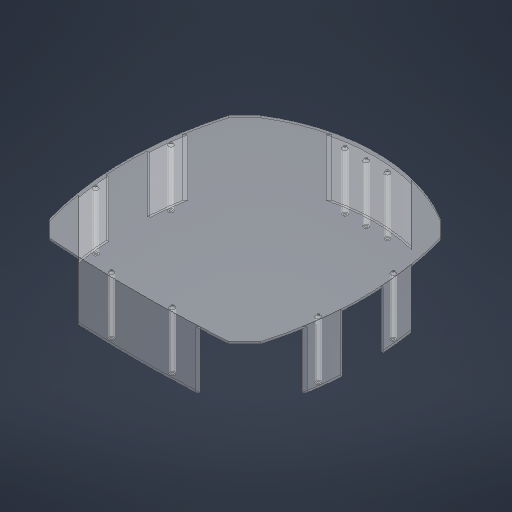
# Autodesk Inventor part: Spider_Robot_Chasis_Top_V1
Saved by Autodesk Inventor 2026.2 (Build 302298010, 298A)
## iProperties
Created: 2026-09-09
Part Number: Spider_Robot_Chasis_Top_V1
Material: Generic
Document SubType Name: Modeling
Designer: Entity
Density: 1 g/cm^3
Appearance: Clear - Light
Mass: 138.389 g
Surface Area: 1463.19 cm^2
Volume: 138.389 cm^3
Author: Entity
Autodesk Inventor part; units mm, degrees
ref_plane "YZ Plane" through (0, 0, 0) normal (1, 0, 0) x (0, 1, 0)
ref_plane "XZ Plane" through (0, 0, 0) normal (0, 1, 0) x (-1, 0, 0)
ref_plane "XY Plane" through (0, 0, 0) normal (0, 0, 1) x (1, 0, 0)
sketch "Sketch1" plane through (0, 0, 0) normal (0, 1, 0) x (-1, 0, 0)
  line L0 (11.257, 34.2721) -> (-44.743, 34.2721)
  line L1 (-44.743, 34.2721) -> (-44.743, -50.7279)
  line L2 (-44.743, -50.7279) -> (11.257, -50.7279)
  line L3 (11.257, -50.7279) -> (11.257, 34.2721)
  line L4 (-16.743, -50.7279) -> (-16.743, -57.7279)
  line L5 (14.507, -57.7279) -> (-47.993, -57.7279)
  line L6 (-47.993, -57.7279) -> (-47.993, -83.1279)
  line L7 (-47.993, -83.1279) -> (14.507, -83.1279)
  line L8 (14.507, -83.1279) -> (14.507, -57.7279)
  line L9 (-16.743, 34.2721) -> (-16.743, 41.2721)
  line L10 (-4.243, 41.2721) -> (-29.243, 41.2721)
  line L11 (-29.243, 41.2721) -> (-29.243, 51.2721)
  line L12 (-29.243, 51.2721) -> (-4.243, 51.2721)
  line L13 (-4.243, 51.2721) -> (-4.243, 41.2721)
  line L14 (-16.743, -83.1279) -> (-16.743, -90.1279)
  line L15 (23.257, -160.1279) -> (-56.743, -160.1279)
  line L16 (-56.743, -160.1279) -> (-56.743, -90.1279)
  line L17 (-56.743, -90.1279) -> (23.257, -90.1279)
  line L18 (23.257, -90.1279) -> (23.257, -160.1279)
  line L19 (14.507, -54.4279) -> (21.507, -54.4279)
  line L20 (14.507, -57.7279) -> (14.507, -54.4279)
  line L21 (46.907, -85.6779) -> (21.507, -85.6779)
  line L22 (21.507, -85.6779) -> (21.507, -23.1779)
  line L23 (21.507, -23.1779) -> (46.907, -23.1779)
  line L24 (46.907, -23.1779) -> (46.907, -85.6779)
  line L25 (-80.393, -85.6779) -> (-54.993, -85.6779)
  line L26 (-54.993, -85.6779) -> (-54.993, -23.1779)
  line L27 (-54.993, -23.1779) -> (-80.393, -23.1779)
  line L28 (-80.393, -23.1779) -> (-80.393, -85.6779)
  line L29 (-80.393, -54.4279) -> (-87.393, -54.4279)
  line L30 (-16.743, -160.1279) -> (-16.743, 51.2721)
  line L31 (-16.743, -54.4279) -> (63.257, -54.4279) construction
  line L32 (-16.743, -54.4279) -> (-69.7761, -107.4609)
  line L33 (-16.743, -54.4279) -> (58.257, -54.4279) construction
  line L34 (-69.7761, -107.4609) -> (-80.3827, -118.0675)
  line L35 (-80.3827, -118.0675) -> (-88.1608, -110.2893)
  line L36 (-88.1608, -110.2893) -> (-119.2735, -141.402)
  line L37 (-119.2735, -141.402) -> (-103.7172, -156.9584)
  line L38 (-103.7172, -156.9584) -> (-72.6045, -125.8457)
  line L39 (-72.6045, -125.8457) -> (-80.3827, -118.0675)
  line L40 (86.0976, -54.4279) -> (-151.9015, -54.4279)
  line L41 (-87.393, -54.4279) -> (-87.393, -65.4279)
  line L42 (-87.393, -65.4279) -> (-131.393, -65.4279)
  line L43 (-131.393, -65.4279) -> (-131.393, -43.4279)
  line L44 (-131.393, -43.4279) -> (-87.393, -43.4279)
  line L45 (-87.393, -43.4279) -> (-87.393, -54.4279)
  line L46 (-80.3827, 9.2117) -> (-88.1608, 1.4335)
  line L47 (-88.1608, 1.4335) -> (-119.2735, 32.5462)
  line L48 (-119.2735, 32.5462) -> (-103.7172, 48.1026)
  line L49 (-103.7172, 48.1026) -> (-72.6045, 16.9899)
  line L50 (-72.6045, 16.9899) -> (-80.3827, 9.2117)
  line L51 (46.8966, -118.0675) -> (54.6747, -110.2893)
  line L52 (54.6747, -110.2893) -> (85.7874, -141.402)
  line L53 (85.7874, -141.402) -> (70.2311, -156.9584)
  line L54 (70.2311, -156.9584) -> (39.1184, -125.8457)
  line L55 (39.1184, -125.8457) -> (46.8966, -118.0675)
  line L56 (53.907, -54.4279) -> (53.907, -65.4279)
  line L57 (53.907, -65.4279) -> (97.907, -65.4279)
  line L58 (97.907, -65.4279) -> (97.907, -43.4279)
  line L59 (97.907, -43.4279) -> (53.907, -43.4279)
  line L60 (53.907, -43.4279) -> (53.907, -54.4279)
  line L61 (54.6747, 1.4335) -> (85.7874, 32.5462)
  line L62 (85.7874, 32.5462) -> (70.2311, 48.1026)
  line L63 (70.2311, 48.1026) -> (39.1184, 16.9899)
  line L64 (46.8966, 9.2117) -> (54.6747, 1.4335)
  line L65 (39.1184, 16.9899) -> (46.8966, 9.2117)
  point P0 (-16.743, -57.7279)
  point P1 (-29.243, 46.2721)
  point P2 (-16.743, -90.1279)
  point P3 (21.507, -54.4279)
  point P4 (-83.893, -54.4279)
  point P5 (-54.993, -54.4279)
  point P6 (-44.743, -8.2279)
  point P7 (-87.393, -42.4279)
  dimension "d22" = 85
  dimension "d23" = 56
  dimension "d29" = 7
  dimension "d30" = 62.5
  dimension "d31" = 25.4
  dimension "d32" = 0
  dimension "d33" = 0
  dimension "d34" = 7
  dimension "d35" = 10
  dimension "d36" = 25
  dimension "d37" = 0
  dimension "d38" = 0
  dimension "d53" = 7
  dimension "d54" = 80
  dimension "d55" = 70
  dimension "d56" = 0
  dimension "d57" = 0
  dimension "d59" = 7
  dimension "d60" = 3.3
  dimension "d61" = 25.4
  dimension "d62" = 62.5
  dimension "d63" = 0
  dimension "d64" = 0
  dimension "d65" = 7
  dimension "d73" = 75
  dimension "d74" = 135
  dimension "d75" = 15
  dimension "d76" = 11
  dimension "d77" = 44
  dimension "d78" = 22
  dimension "d84" = 31.25
  dimension "d85" = 46.2
  dimension "d87" = 25.4
  dimension "d88" = 62.5
  dimension "d91" = 7
  dimension "d92" = 10.25
  dimension "d97" = 11
  dimension "d98" = 44
  dimension "d99" = 22
  constraints: 132 end point, 20 symmetric about line, 15 midpoint, 12 perpendicular, 10 parallel, 9 horizontal, 7 point on line, 5 vertical, 1 equal length
  measures "d22" distance of L0.end L1.end
  measures "d23" distance of L1.end L2.end
  measures "d29" distance of L4.start L4.end
  measures "d30" distance of L6.end L7.end
  measures "d31" distance of L5.end L6.end
  measures "d32" distance of L4.end point (-16.743, -57.728)
  measures "d33" distance of point (-16.743, -57.728) L4.end
  measures "d34" distance of L9.start L9.end
  measures "d35" distance of L12.end L10.start
  measures "d36" distance of L11.end L12.end
  measures "d37" distance of L9.end point (-16.743, 41.272)
  measures "d38" distance of L9.end point (-16.743, 41.272)
  measures "d53" distance of L14.start L14.end
  measures "d54" distance of L16.end L17.end
  measures "d55" distance of L15.end L16.end
  measures "d56" distance of L14.end point (-16.743, -90.128)
  measures "d57" distance of point (-16.743, -90.128) L14.end
  measures "d59" distance of L19.start L19.end
  measures "d60" distance of L5.start L19.start
  measures "d61" distance of L22.end L23.end
  measures "d62" distance of L21.end L22.end
  measures "d63" distance of L19.end point (21.507, -54.428)
  measures "d64" distance of point (21.507, -54.428) L19.end
  measures "d65" distance of L29.start L29.end
  measures "d73" distance of L31.start L32.end
  measures "d74" angle of L32 L33
  measures "d75" distance of L32.end L34.end
  measures "d76" distance of L34.end L35.end
  measures "d77" distance of L35.end L36.end
  measures "d78" distance of L36.end L37.end
  measures "d84" vertical distance of L28.start point (-83.893, -54.428)
  measures "d85" vertical distance of point (-54.993, -54.428) point (-44.743, -8.228)
  measures "d87" distance of L27.start L28.start
  measures "d88" distance of L25.end L27.start
  measures "d91" horizontal distance of L25.end L6.end
  measures "d92" horizontal distance of L27.start point (-44.743, -8.228)
  measures "d97" distance of L29.end L41.end
  measures "d98" distance of L41.end L42.end
  measures "d99" distance of L42.end L43.end
extrude "Extrusion1" add sketch "Sketch1" along normal blind 54 contours L3 L2 L30 L0 | L30 L2 L1 L0 | L30 L7 L32 L5 | L5 L8 L7 L30 | L32 L7 L6 L5 | L30 L15 L16 L32 L17 | L17 L18 L15 L30 | L32 L16 L17 | L10 L30 L12 L13 | L10 L11 L12 L30 | L21 L22 L40 L24 | L40 L22 L23 L24 | L28 L40 L26 L25 | L28 L27 L26 L40 | L39 L38 L37 L36 L35 | L41 L42 L43 L40 | L40 L43 L44 L45 | L46 L47 L48 L49 L50 | L51 L52 L53 L54 L55 | L60 L59 L58 L57 L56 | L64 L65 L63 L62 L61
sketch "Sketch2" plane through (0, 0, 0) normal (0, -1, 0) x (1, 0, 0)
  line L0 (56.743, -160.1279) -> (-23.257, -160.1279) projected
  line L1 (4.243, 51.2721) -> (29.243, 51.2721) projected
  line L2 (-85.7874, 32.5462) -> (-70.2311, 48.1026) projected
  line L3 (-70.2311, 48.1026) -> (-229.2278, -110.8941)
  line L4 (-70.2311, -156.9584) -> (-85.7874, -141.402) projected
  line L5 (-70.2311, -156.9584) -> (-201.5199, -25.6696)
  line L6 (103.7172, -156.9584) -> (72.6045, -125.8457) projected
  line L7 (103.7172, -156.9584) -> (295.0011, 34.3256)
  line L8 (103.7172, 48.1026) -> (119.2735, 32.5462) projected
  line L9 (103.7172, 48.1026) -> (277.6654, -125.8457)
  line L10 (103.7172, 48.1026) -> (-70.2311, 48.1026)
  arc A0 (-70.2311, -156.9584) -> (103.7172, -156.9584) centre (16.743, -16.5068) ccw
  line L11 (47.993, -83.1279) -> (-14.507, -83.1279) projected
  line L12 (16.743, -83.1279) -> (16.743, -57.7279)
  line L13 (-14.507, -57.7279) -> (47.993, -57.7279) projected
  arc A1 (103.7172, 48.1026) -> (-70.2311, 48.1026) centre (16.743, -1143.6334) ccw
  line L14 (-97.907, -65.4279) -> (-97.907, -43.4279) projected
  arc A2 (-85.7874, 32.5462) -> (-85.7874, -141.402) centre (215.2401, -54.4279) ccw
  line L15 (131.393, -43.4279) -> (131.393, -65.4279) projected
  arc A3 (119.2735, -141.402) -> (119.2735, 32.5462) centre (-181.754, -54.4279) ccw
  point P0 (0, 0)
  point P1 (-172.7616, -54.4279)
  dimension "d133" = 1194.9055
  dimension "d134" = 313.3402
  dimension "d135" = 313.3402
  dimension "d136" = 165.2003
  constraints: 12 end point, 10 point on circle, 4 centre point, 3 collinear, 2 midpoint, 1 horizontal, 1 perpendicular, 1 point on line
  measures "d133" radius of A1
  measures "d134" radius of A3
  measures "d135" radius of A2
  measures "d136" radius of A0
extrude "Extrusion2" add sketch "Sketch2" along normal blind 57 contours L2 L10 L8 A3 L15 L7 A0 L4 A2 L14 | A1 L10 | L14 A2 | A3 L15
sketch "Sketch11" plane through (0, 54, 0) normal (0, 1, 0) x (1, 0, 0)
  line L0 (56.743, 160.1279) -> (-23.257, 160.1279) projected
  line L1 (56.743, 90.1279) -> (56.743, 160.1279) projected
  line L2 (-23.257, 160.1279) -> (56.743, 160.1279)
  line L3 (56.743, 160.1279) -> (56.743, 90.1279)
  line L4 (56.743, 90.1279) -> (-23.257, 90.1279)
  line L5 (-23.257, 90.1279) -> (-23.257, 160.1279)
  line L6 (47.993, 83.1279) -> (-14.507, 83.1279) projected
  line L7 (-14.507, 57.7279) -> (47.993, 57.7279) projected
  line L8 (-14.507, 83.1279) -> (47.993, 83.1279)
  line L9 (47.993, 83.1279) -> (47.993, 57.7279)
  line L10 (47.993, 57.7279) -> (-14.507, 57.7279)
  line L11 (-14.507, 57.7279) -> (-14.507, 83.1279)
  line L12 (-21.507, 85.6779) -> (-46.907, 85.6779) projected
  line L13 (-21.507, 23.1779) -> (-21.507, 85.6779) projected
  line L14 (-46.907, 85.6779) -> (-21.507, 85.6779)
  line L15 (-21.507, 85.6779) -> (-21.507, 23.1779)
  line L16 (-21.507, 23.1779) -> (-46.907, 23.1779)
  line L17 (-46.907, 23.1779) -> (-46.907, 85.6779)
  line L18 (80.393, 23.1779) -> (80.393, 85.6779) projected
  line L19 (54.993, 23.1779) -> (80.393, 23.1779)
  line L20 (80.393, 23.1779) -> (80.393, 85.6779)
  line L21 (80.393, 85.6779) -> (54.993, 85.6779)
  line L22 (54.993, 85.6779) -> (54.993, 23.1779)
  line L23 (44.743, 50.7279) -> (-11.257, 50.7279) projected
  line L24 (-11.257, -34.2721) -> (44.743, -34.2721) projected
  line L25 (-11.257, 50.7279) -> (44.743, 50.7279)
  line L26 (44.743, 50.7279) -> (44.743, -34.2721)
  line L27 (44.743, -34.2721) -> (-11.257, -34.2721)
  line L28 (-11.257, -34.2721) -> (-11.257, 50.7279)
  line L29 (29.243, -41.2721) -> (4.243, -41.2721) projected
  line L30 (29.243, -51.2721) -> (29.243, -41.2721) projected
  line L31 (4.243, -41.2721) -> (29.243, -41.2721)
  line L32 (29.243, -41.2721) -> (29.243, -51.2721)
  line L33 (29.243, -51.2721) -> (4.243, -51.2721)
  line L34 (4.243, -51.2721) -> (4.243, -41.2721)
  line L35 (-54.6747, 110.2893) -> (-39.1184, 125.8457) projected
  line L36 (-54.6747, 110.2893) -> (-39.1184, 125.8457)
  line L37 (-39.1184, 125.8457) -> (-70.2311, 156.9584)
  line L38 (-85.7874, 141.402) -> (-54.6747, 110.2893)
  line L39 (103.7172, 156.9584) -> (72.6045, 125.8457) projected
  line L40 (103.7172, 156.9584) -> (72.6045, 125.8457)
  line L41 (88.1608, 110.2893) -> (119.2735, 141.402) projected
  line L42 (72.6045, 125.8457) -> (88.1608, 110.2893)
  line L43 (88.1608, 110.2893) -> (119.2735, 141.402)
  line L44 (119.2735, 141.402) -> (103.7172, 156.9584)
  line L45 (-39.1184, -16.9899) -> (-54.6747, -1.4335) projected
  line L46 (-54.6747, -1.4335) -> (-39.1184, -16.9899)
  line L47 (-39.1184, -16.9899) -> (-70.2311, -48.1026)
  line L48 (-70.2311, -48.1026) -> (-85.7874, -32.5462)
  line L49 (-85.7874, -32.5462) -> (-54.6747, -1.4335)
  line L50 (88.1608, -1.4335) -> (72.6045, -16.9899) projected
  line L51 (72.6045, -16.9899) -> (88.1608, -1.4335)
  line L52 (103.7172, -48.1026) -> (119.2735, -32.5462) projected
  line L53 (88.1608, -1.4335) -> (119.2735, -32.5462)
  line L54 (119.2735, -32.5462) -> (103.7172, -48.1026)
  line L55 (103.7172, -48.1026) -> (72.6045, -16.9899)
  line L56 (-85.7874, 141.402) -> (-70.2311, 156.9584) projected
  line L57 (-85.7874, 141.402) -> (-70.2311, 156.9584)
  point P0 (0, 0)
  point P1 (87.393, 65.4279)
  point P2 (131.393, 43.4279)
  point P3 (-53.907, 43.4279)
  point P4 (-53.907, 65.4279)
  point P5 (-97.907, 43.4279)
  constraints: 80 end point, 17 equal length, 15 perpendicular, 6 horizontal, 1 point on line
extrude "Extrusion11" cut sketch "Sketch11" against normal blind 54
shell "Shell1" thickness 2 removed faces 1 at (16.743, -57, -33.8711)
sketch "Sketch12" plane through (103.7172, -57, 48.1026) normal (0.7071068, 0, 0.7071068) x (0.7071068, 0, -0.7071068)
  line L0 (22, 57) -> (22, 0) projected
  line L1 (22, 0) -> (0, 0)
  line L2 (0, 0) -> (0, 54)
  line L3 (0, 54) -> (22, 54)
  line L4 (22, 54) -> (22, 0)
  line L5 (11, 54) -> (11, 47)
  point P0 (-39.3255, 57)
  point P1 (22, 54)
  dimension "d140" = 22
  dimension "d141" = 54
  dimension "d144" = 7
  constraints: 10 end point, 3 parallel, 1 horizontal, 1 midpoint, 1 perpendicular
  measures "d140" distance of L2.end L3.end
  measures "d141" distance of L1.end L2.end
  measures "d144" distance of L5.start L5.end
extrude "Extrusion12" cut sketch "Sketch12" against normal blind 57
sketch "Sketch13" plane through (0, 0, 0) normal (0, 1, 0) x (1, 0, 0)
  line L0 (119.2735, -32.5462) -> (103.7172, -48.1026) projected
  line L1 (111.4954, -40.3244) -> (97.3532, -54.4665)
  line L2 (97.3532, -54.4665) -> (83.2111, -40.3244)
  line L3 (83.2111, -40.3244) -> (105.1314, -18.4041)
  line L4 (103.7172, -48.1026) -> (89.575, -33.9605)
  line L5 (119.2735, -32.5462) -> (105.1314, -18.4041)
  line L6 (83.2111, -40.3244) -> (65.4164, -58.1191)
  line L7 (65.4164, -58.1191) -> (143.1792, 19.6438)
  arc A0 (119.2735, -32.5462) -> (119.2735, 141.402) centre (-181.754, 54.4279) ccw projected
  arc A1 (119.2735, -32.5462) -> (127.4951, 3.9596) centre (-181.754, 54.4279) ccw
  arc A2 (-70.2311, -48.1026) -> (103.7172, -48.1026) centre (16.743, 1143.6334) ccw projected
  arc A3 (73.6177, -49.9178) -> (103.7172, -48.1026) centre (16.743, 1143.6334) ccw
  line L8 (16.743, 179.7071) -> (16.743, 16.5068)
  line L9 (-85.7874, -32.5462) -> (-70.2311, -48.1026)
  line L10 (-78.0093, -40.3244) -> (-63.8671, -54.4665)
  line L11 (-63.8671, -54.4665) -> (-49.725, -40.3244)
  line L12 (-70.2311, -48.1026) -> (-56.089, -33.9605)
  line L13 (-85.7874, -32.5462) -> (-71.6453, -18.4041)
  line L14 (-31.9303, -58.1191) -> (-109.6932, 19.6438)
  arc A4 (-85.7874, 141.402) -> (-85.7874, -32.5462) centre (215.2401, 54.4279) ccw
  arc A5 (-70.2311, -48.1026) -> (103.7172, -48.1026) centre (16.743, 1143.6334) ccw
  line L15 (87.393, 65.4279) -> (87.393, 43.4279) projected
  line L16 (87.393, 54.4279) -> (-53.907, 54.4279)
  line L17 (-53.907, 43.4279) -> (-53.907, 65.4279) projected
  line L18 (97.3532, 163.3223) -> (83.2111, 149.1802)
  line L19 (103.7172, 156.9584) -> (89.575, 142.8162)
  line L20 (119.2735, 141.402) -> (105.1314, 127.2599)
  line L21 (65.4164, 166.9749) -> (143.1792, 89.212)
  line L22 (-31.9303, 166.9749) -> (-109.6932, 89.212)
  line L23 (-70.2311, 156.9584) -> (-56.089, 142.8162)
  line L24 (-85.7874, 141.402) -> (-71.6453, 127.2599)
  line L25 (-63.8671, 163.3223) -> (-49.725, 149.1802)
  line L26 (119.2735, 141.402) -> (103.7172, 156.9584)
  line L27 (65.4164, 166.9749) -> (53.4842, 178.9071)
  line L28 (-31.9303, 166.9749) -> (-12.9219, 185.9833)
  line L29 (-85.7874, 141.402) -> (-70.2311, 156.9584)
  line L30 (-84.0084, 140.3527) -> (-68.9814, 155.3796) projected
  arc A6 (103.7172, 156.9584) -> (-70.2311, 156.9584) centre (16.743, 16.5068) ccw projected
  arc A7 (103.7172, 156.9584) -> (55.2299, 177.1614) centre (16.743, 16.5068) ccw
  arc A8 (-21.7438, 177.1614) -> (-70.2311, 156.9584) centre (16.743, 16.5068) ccw
  point P0 (0, 0)
  point P1 (73.6177, -49.9178)
  point P2 (-94.009, 3.9596)
  point P3 (-70.2311, -48.1026)
  point P4 (-40.1316, -49.9178)
  point P5 (127.4951, 104.8962)
  point P6 (-21.7438, 177.1614)
  point P7 (-94.009, 104.8962)
  dimension "d145" = 20
  dimension "d146" = 20
  constraints: 54 end point, 26 symmetric about line, 16 point on circle, 6 centre point, 6 point on line, 3 midpoint, 3 parallel, 1 collinear, 1 concentric, 1 perpendicular, 1 vertical, 2 other
  measures "d145" distance of L1.start L1.end
  measures "d146" distance of L1.end L2.end
extrude "Extrusion13" cut sketch "Sketch13" against normal blind 57 contours L0 L4 L3 L5 | L5 L7 A0 | A2 L2 L3 L4 | L21 L20 A0 | A2 L6 L2 | L20 L21 L19 L26 | L19 L21 L18 A6 | A2 L11 L14 | L18 L21 L27 A6 | A2 L12 L14 L11 | L9 L13 L14 L12 | L28 L22 L25 A6 | L13 A4 L14 | L25 L22 L23 A6 | L23 L22 L24 L29 | A4 L24 L22
sketch "Sketch15" plane through (0, 54, 0) normal (0, 1, 0) x (1, 0, 0)
  line L0 (131.393, 65.4279) -> (87.393, 65.4279) projected
  line L1 (87.393, 43.4279) -> (131.393, 43.4279) projected
  line L2 (87.393, 65.4279) -> (131.393, 65.4279)
  line L3 (131.393, 65.4279) -> (131.393, 43.4279)
  line L4 (131.393, 43.4279) -> (87.393, 43.4279)
  line L5 (87.393, 43.4279) -> (87.393, 65.4279)
  line L6 (-53.907, 43.4279) -> (-53.907, 65.4279) projected
  line L7 (-97.907, 43.4279) -> (-53.907, 43.4279) projected
  line L8 (-53.907, 65.4279) -> (-97.907, 65.4279)
  line L9 (-97.907, 65.4279) -> (-97.907, 43.4279)
  line L10 (-97.907, 43.4279) -> (-53.907, 43.4279)
  line L11 (-53.907, 43.4279) -> (-53.907, 65.4279)
  line L12 (-97.907, 65.4279) -> (-97.907, 43.4279) projected
  circle A0 centre (-97.907, 54.4279) radius 20
  line L13 (-53.907, 43.4279) -> (-93.7044, 34.8744)
  line L14 (-53.907, 65.4279) -> (-93.7044, 73.9814)
  arc A1 (55.2299, 177.1614) -> (-21.7438, 177.1614) centre (16.743, 16.5068) ccw projected
  circle A2 centre (131.393, 54.4279) radius 20
  line L15 (87.393, 43.4279) -> (127.1905, 34.8744)
  line L16 (87.393, 65.4279) -> (127.1905, 73.9814)
  point P0 (0, 0)
  dimension "d153" = 40
  constraints: 24 end point, 4 parallel, 4 point on circle, 2 centre point, 2 horizontal, 2 perpendicular, 2 tangent, 1 midpoint
  measures "d153" diameter of A0
extrude "Extrusion15" cut sketch "Sketch15" against normal blind 170
sketch "Sketch16" plane through (0, 0, 0) normal (0, 1, 0) x (1, 0, 0)
  arc A0 (55.2299, 177.1614) -> (-21.7438, 177.1614) centre (16.743, 16.5068) ccw projected
  line L0 (16.743, 16.5068) -> (16.743, 181.7071)
  circle A1 centre (16.743, 16.5068) radius 165.2003
  arc A2 (-94.009, 104.8962) -> (-97.4615, 74.4229) centre (215.2401, 54.4279) ccw projected
  circle A3 centre (215.2401, 54.4279) radius 313.3402
  arc A4 (130.9476, 74.4229) -> (127.4951, 104.8962) centre (-181.754, 54.4279) ccw projected
  circle A5 centre (-181.754, 54.4279) radius 313.3402
  arc A6 (-40.1316, -49.9178) -> (73.6177, -49.9178) centre (16.743, 1143.6334) ccw projected
  circle A7 centre (16.743, 1143.6334) radius 1194.9055
  line L1 (16.743, 181.7071) -> (103.7174, 156.9583)
  line L2 (103.7174, 156.9583) -> (117.4581, 147.4557)
  line L3 (-98.1001, 54.4279) -> (-85.7875, -32.5459)
  line L4 (-85.7875, -32.5459) -> (-70.2315, -48.1026)
  line L5 (103.7174, 156.9583) -> (119.2736, 141.4018)
  line L6 (16.743, 181.7071) -> (-70.2313, 156.9583)
  line L7 (131.5862, 54.4279) -> (119.2736, -32.5459)
  line L8 (119.2736, -32.5459) -> (103.7176, -48.1026)
  line L9 (-70.2313, 156.9583) -> (-85.7875, 141.4018)
  point P0 (0, 0)
  point P1 (127.4951, 104.8962)
  point P2 (55.2299, 177.1614)
  point P3 (-21.7438, 177.1614)
  point P4 (-94.009, 104.8962)
  point P5 (-97.4615, 74.4229)
  point P6 (73.6177, -49.9178)
  dimension "d154" = 90.427
  dimension "d155" = 87.841
  dimension "d156" = 22
  dimension "d157" = 22
  constraints: 20 end point, 8 point on circle, 5 symmetric about line, 4 coincident, 3 centre point, 1 vertical, 3 other
  measures "d154" distance of L0.end L1.end
  measures "d155" distance of L3.start L3.end
  measures "d156" distance of L3.end L4.end
  measures "d157" distance of L1.end L5.end
extrude "Extrusion16" add sketch "Sketch16" against normal blind 2 contours A1 L1 A0 | L6 A1 A0 | L1 L5 A5 A4 L7 L8 A7 A6 L4 L3 A3 A2 L9 L6 | A5 L7 | A3 L3
sketch "Sketch17" plane through (16.743, -2, -1143.6334) normal (0, -1, 0) x (1, 0, 0)
  line L0 (-58.9793, 1191.4466) -> (58.9793, 1191.4466)
  line L1 (58.9793, 1191.4466) -> (0, 1191.4466)
  line L2 (0, 1191.4466) -> (29.4896, 1191.4466)
  line L3 (0, 1191.4466) -> (-58.9793, 1191.4466)
  line L4 (-29.4896, 1191.4466) -> (-29.4896, 1188.9466)
  circle A0 centre (-29.4896, 1188.9466) radius 2.5
  circle A1 centre (29.4896, 1188.9466) radius 2.5
  line L5 (-108.3152, 1142.1106) -> (-112.2097, 1109.056)
  line L6 (-112.2097, 1109.056) -> (-110.2624, 1125.5833)
  line L7 (-112.2097, 1069.3549) -> (-108.3152, 1036.3003)
  line L8 (-108.3152, 1036.3003) -> (-110.2624, 1052.8276)
  line L9 (-110.2624, 1125.5833) -> (-107.7796, 1125.8759)
  circle A2 centre (-107.7796, 1125.8759) radius 2.5
  line L10 (-112.2097, 1069.3549) -> (-110.2624, 1052.8276)
  line L11 (-110.2624, 1052.8276) -> (-107.7796, 1053.1202)
  circle A3 centre (-107.7796, 1053.1202) radius 2.5
  line L12 (41.2368, 969.222) -> (-41.2368, 969.222)
  line L13 (-41.2368, 969.222) -> (0, 969.222)
  line L14 (0, 969.222) -> (0, 971.722)
  circle A4 centre (0, 971.722) radius 2.5
  line L15 (0, 969.222) -> (41.2368, 969.222)
  line L16 (41.2368, 969.222) -> (20.6184, 969.222)
  line L17 (20.6184, 969.222) -> (20.6184, 971.722)
  circle A5 centre (20.6184, 971.722) radius 2.5
  line L18 (-41.2368, 969.222) -> (-20.6184, 969.222)
  line L19 (-20.6184, 969.222) -> (-20.6184, 971.722)
  circle A6 centre (-20.6184, 971.722) radius 2.5
  circle A7 centre (107.7796, 1125.8759) radius 2.5
  circle A8 centre (107.7796, 1053.1202) radius 2.5
  dimension "d160" = 2.5
  dimension "d161" = 2.5
  dimension "d162" = 2.5
  dimension "d163" = 2.5
  dimension "d164" = 2.5
  constraints: 40 end point, 8 midpoint, 6 coincident, 5 vertical alignment, 4 perpendicular, 3 horizontal, 2 centre point, 2 collinear, 2 symmetric about line, 2 vertical, 18 other
  measures "d160" distance of L4.start L4.end
  measures "d161" distance of L6.end L9.end
  measures "d162" distance of L8.end L11.end
  measures "d163" distance of L13.end L14.end
  measures "d164" distance of L16.end L17.end
extrude "Extrusion17" add sketch "Sketch17" along normal blind 55
sketch "Sketch18" plane through (-12.7466, -57, 45.3132) normal (0, -1, 0) x (1, 0, 0)
  circle A0 centre (0, 0) radius 2.5 projected
  circle A1 centre (58.9793, 0) radius 2.5 projected
  circle A2 centre (137.2692, -63.0707) radius 2.5 projected
  circle A3 centre (137.2692, -135.8264) radius 2.5 projected
  circle A4 centre (29.4896, -217.2246) radius 2.5 projected
  circle A5 centre (50.108, -217.2246) radius 2.5 projected
  circle A6 centre (8.8712, -217.2246) radius 2.5 projected
  circle A7 centre (-78.29, -135.8264) radius 2.5 projected
  circle A8 centre (-78.29, -63.0707) radius 2.5 projected
  point P0 (12.7466, -45.3132)
  constraints: 9 coincident
hole "Hole1" at (124.5227, -57, -90.5132) at (-91.0366, -57, -17.7575) at (124.5227, -57, -17.7575) at (46.2327, -57, 45.3132) at (-12.7466, -57, 45.3132) at (-91.0366, -57, -90.5132) at (-3.8754, -57, -171.9114) at (16.743, -57, -171.9114) at (37.3615, -57, -171.9114) direction (0, 1, 0) diameter 2.459 end through all thread size "M3x0.5" class "6H" standard "ISO Metric profile"
sketch "Sketch3" plane through (0, 54, 0) normal (0, 1, 0) x (1, 0, 0)
  line L0 (131.393, 43.4279) -> (131.393, 65.4279) projected
  line L1 (131.393, 54.4279) -> (87.393, 54.4279)
  line L2 (87.393, 65.4279) -> (87.393, 43.4279) projected
  line L3 (87.393, 54.4279) -> (88.393, 54.4279)
  line L4 (88.393, 54.4279) -> (88.393, 43.4279)
  line L5 (87.393, 43.4279) -> (131.393, 43.4279) projected
  line L6 (88.393, 43.4279) -> (88.393, 44.4279)
  line L7 (88.393, 44.4279) -> (130.393, 44.4279)
  line L8 (130.393, 44.4279) -> (130.393, 64.4279)
  line L9 (130.393, 64.4279) -> (88.393, 64.4279)
  line L10 (88.393, 64.4279) -> (88.393, 54.4279)
  line L11 (103.7172, -48.1026) -> (119.2735, -32.5462) projected
  line L12 (111.4954, -40.3244) -> (80.3827, -9.2117)
  line L13 (88.1608, -1.4335) -> (72.6045, -16.9899) projected
  line L14 (111.4954, -40.3244) -> (110.7882, -39.6173)
  line L15 (110.7882, -39.6173) -> (117.8593, -32.5462)
  line L16 (119.2735, -32.5462) -> (88.1608, -1.4335) projected
  line L17 (103.6075, -46.5778) -> (110.7882, -39.6173)
  line L18 (103.6075, -46.5778) -> (73.312, -16.2824)
  line L19 (117.8593, -32.5462) -> (88.1608, -2.8478)
  line L20 (88.1608, -2.8478) -> (74.0191, -16.9895)
  line L21 (110.7882, 148.4731) -> (117.8593, 141.402)
  line L22 (103.6075, 155.4336) -> (110.7882, 148.4731)
  line L23 (103.6075, 155.4336) -> (73.312, 125.1381)
  line L24 (117.8593, 141.402) -> (88.1608, 111.7035)
  line L25 (88.1608, 111.7035) -> (74.0191, 125.8453)
  line L26 (-54.907, 54.4279) -> (-54.907, 43.4279)
  line L27 (-54.907, 44.4279) -> (-96.907, 44.4279)
  line L28 (-96.907, 44.4279) -> (-96.907, 64.4279)
  line L29 (-96.907, 64.4279) -> (-54.907, 64.4279)
  line L30 (-54.907, 64.4279) -> (-54.907, 54.4279)
  line L31 (-77.3022, -39.6173) -> (-84.3732, -32.5462)
  line L32 (-70.1214, -46.5778) -> (-77.3022, -39.6173)
  line L33 (-70.1214, -46.5778) -> (-39.8259, -16.2824)
  line L34 (-84.3732, -32.5462) -> (-54.6747, -2.8478)
  line L35 (-54.6747, -2.8478) -> (-40.533, -16.9895)
  line L36 (-54.6747, 111.7035) -> (-40.533, 125.8453)
  line L37 (-70.1214, 155.4336) -> (-39.8259, 125.1381)
  line L38 (-84.3732, 141.402) -> (-54.6747, 111.7035)
  line L39 (-70.1214, 155.4336) -> (-77.3022, 148.4731)
  line L40 (-77.3022, 148.4731) -> (-84.3732, 141.402)
  point P0 (0, 0)
  dimension "d100" = 1
  dimension "d101" = 1
  dimension "d102" = 42
  dimension "d103" = 20
  dimension "d104" = 1
  dimension "d105" = 10
  dimension "d109" = 42
  constraints: 70 end point, 10 point on line, 8 perpendicular, 4 midpoint, 1 horizontal
  measures "d100" distance of L1.end L3.end
  measures "d101" distance of L4.end L6.end
  measures "d102" distance of L6.end L7.end
  measures "d103" distance of L7.end L8.end
  measures "d104" distance of L12.start L14.end
  measures "d105" distance of L14.end L15.end
  measures "d109" distance of L15.end L19.end
sketch "Sketch4" plane through (0, 54, 0) normal (0, 1, 0) x (1, 0, 0)
  line L0 (103.7172, -48.1026) -> (119.2735, -32.5462) projected
  line L1 (119.2735, -32.5462) -> (88.1608, -1.4335) projected
  line L2 (103.7172, -48.1026) -> (119.2735, -32.5462)
  line L3 (119.2735, -32.5462) -> (88.1608, -1.4335)
  line L4 (88.1608, -1.4335) -> (72.6045, -16.9899)
  line L5 (72.6045, -16.9899) -> (103.7172, -48.1026)
  line L6 (87.393, 43.4279) -> (131.393, 43.4279) projected
  line L7 (131.393, 43.4279) -> (87.393, 43.4279)
  line L8 (87.393, 65.4279) -> (87.393, 43.4279) projected
  line L9 (87.393, 43.4279) -> (87.393, 65.4279)
  line L10 (87.393, 65.4279) -> (131.393, 65.4279)
  line L11 (131.393, 65.4279) -> (131.393, 43.4279)
  line L12 (130.393, 64.4279) -> (130.393, 44.4279) projected
  line L13 (56.743, 160.1279) -> (-23.257, 160.1279) projected
  line L14 (4.243, -51.2721) -> (29.243, -51.2721) projected
  line L15 (103.7172, 156.9584) -> (119.2735, 141.402)
  line L16 (119.2735, 141.402) -> (88.1608, 110.2893)
  line L17 (88.1608, 110.2893) -> (72.6045, 125.8457)
  line L18 (72.6045, 125.8457) -> (103.7172, 156.9584)
  line L19 (-70.2311, -48.1026) -> (-85.7874, -32.5462)
  line L20 (-85.7874, -32.5462) -> (-54.6747, -1.4335)
  line L21 (-54.6747, -1.4335) -> (-39.1184, -16.9899)
  line L22 (-39.1184, -16.9899) -> (-70.2311, -48.1026)
  line L23 (-53.907, 43.4279) -> (-97.907, 43.4279)
  line L24 (-97.907, 43.4279) -> (-53.907, 43.4279)
  line L25 (-53.907, 65.4279) -> (-53.907, 43.4279)
  line L26 (-53.907, 43.4279) -> (-53.907, 65.4279)
  line L27 (-53.907, 65.4279) -> (-97.907, 65.4279)
  line L28 (-97.907, 65.4279) -> (-97.907, 43.4279)
  line L29 (-96.907, 64.4279) -> (-96.907, 44.4279)
  line L30 (-39.1184, 125.8457) -> (-70.2311, 156.9584)
  line L31 (-54.6747, 110.2893) -> (-39.1184, 125.8457)
  line L32 (-85.7874, 141.402) -> (-54.6747, 110.2893)
  line L33 (-70.2311, 156.9584) -> (-85.7874, 141.402)
  point P0 (0, 0)
  constraints: 54 end point, 4 perpendicular, 3 collinear, 1 parallel
sketch "Sketch5" plane through (0, 54, 0) normal (0, 1, 0) x (1, 0, 0)
  line L0 (56.743, 160.1279) -> (-23.257, 160.1279) projected
  line L1 (16.743, 160.1279) -> (16.743, 90.1279)
  line L2 (-23.257, 90.1279) -> (56.743, 90.1279) projected
  line L3 (16.743, 160.1279) -> (16.743, 157.6279)
  line L4 (16.743, 157.6279) -> (54.243, 157.6279)
  line L5 (54.243, 157.6279) -> (54.243, 92.6279)
  line L6 (54.243, 92.6279) -> (16.743, 92.6279)
  line L7 (16.743, 92.6279) -> (-20.757, 92.6279)
  line L8 (-20.757, 92.6279) -> (-20.757, 157.6279)
  line L9 (-20.757, 157.6279) -> (16.743, 157.6279)
  point P0 (0, 0)
  dimension "d115" = 2.5
  dimension "d116" = 37.5
  dimension "d117" = 65
  dimension "d118" = 37.5
  constraints: 16 end point, 3 perpendicular, 3 point on line, 2 midpoint, 1 collinear, 1 horizontal
  measures "d115" distance of L1.start L3.end
  measures "d116" distance of L3.end L4.end
  measures "d117" distance of L4.end L5.end
  measures "d118" distance of L6.end L7.end
sketch "Sketch6" plane through (0, -23, 0) normal (0, -1, 0) x (1, 0, 0)
  line L0 (-20.757, -157.6279) -> (54.243, -157.6279) projected
  line L1 (-20.757, -157.6279) -> (-20.757, -92.6279) projected
  line L2 (54.243, -157.6279) -> (-20.757, -157.6279)
  line L3 (-20.757, -157.6279) -> (-20.757, -92.6279)
  line L4 (-20.757, -92.6279) -> (54.243, -92.6279)
  line L5 (54.243, -92.6279) -> (54.243, -157.6279)
  point P0 (0, 0)
  constraints: 8 end point, 2 parallel, 1 horizontal, 1 perpendicular
sketch "Sketch7" plane through (0, 54, 0) normal (0, 1, 0) x (1, 0, 0)
  line L0 (4.243, -41.2721) -> (4.243, -51.2721) projected
  line L1 (29.243, -51.2721) -> (29.243, -41.2721) projected
  line L2 (4.243, -41.2721) -> (29.243, -41.2721)
  line L3 (29.243, -41.2721) -> (29.243, -51.2721)
  line L4 (29.243, -51.2721) -> (4.243, -51.2721)
  line L5 (4.243, -51.2721) -> (4.243, -41.2721)
  point P0 (0, 0)
  constraints: 8 end point, 2 parallel, 1 horizontal, 1 perpendicular
sketch "Sketch8" plane through (0, 54, 0) normal (0, 1, 0) x (1, 0, 0)
  line L0 (44.743, 50.7279) -> (-11.257, 50.7279) projected
  line L1 (-11.257, -34.2721) -> (44.743, -34.2721) projected
  line L2 (-11.257, 50.7279) -> (44.743, 50.7279)
  line L3 (44.743, 50.7279) -> (44.743, -34.2721)
  line L4 (44.743, -34.2721) -> (-11.257, -34.2721)
  line L5 (-11.257, -34.2721) -> (-11.257, 50.7279)
  point P0 (0, 0)
  constraints: 8 end point, 2 parallel, 1 horizontal, 1 perpendicular
sketch "Sketch9" plane through (0, 54, 0) normal (0, 1, 0) x (1, 0, 0)
  line L0 (-21.507, 85.6779) -> (-46.907, 85.6779) projected
  line L1 (-21.507, 23.1779) -> (-21.507, 85.6779) projected
  line L2 (-46.907, 85.6779) -> (-21.507, 85.6779)
  line L3 (-21.507, 85.6779) -> (-21.507, 23.1779)
  line L4 (-21.507, 23.1779) -> (-46.907, 23.1779)
  line L5 (-46.907, 23.1779) -> (-46.907, 85.6779)
  line L6 (80.393, 85.6779) -> (54.993, 85.6779) projected
  line L7 (54.993, 23.1779) -> (80.393, 23.1779) projected
  line L8 (80.393, 85.6779) -> (54.993, 85.6779)
  line L9 (54.993, 85.6779) -> (54.993, 23.1779)
  line L10 (54.993, 23.1779) -> (80.393, 23.1779)
  line L11 (80.393, 23.1779) -> (80.393, 85.6779)
  point P0 (0, 0)
  constraints: 16 end point, 4 parallel, 2 horizontal, 2 perpendicular
sketch "Sketch10" plane through (0, 54, 0) normal (0, 1, 0) x (1, 0, 0)
  line L0 (-14.507, 83.1279) -> (-14.507, 57.7279) projected
  line L1 (47.993, 57.7279) -> (47.993, 83.1279) projected
  line L2 (-14.507, 83.1279) -> (47.993, 83.1279)
  line L3 (47.993, 83.1279) -> (47.993, 57.7279)
  line L4 (47.993, 57.7279) -> (-14.507, 57.7279)
  line L5 (-14.507, 57.7279) -> (-14.507, 83.1279)
  point P0 (0, 0)
  constraints: 8 end point, 2 parallel, 1 horizontal, 1 perpendicular
body "Solid1"
